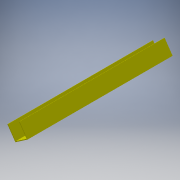
# Autodesk Inventor part: 2018 Concept Hook
Saved by Autodesk Inventor 2018 (Build 220112000, 112)
## iProperties
Created: 2018-01-18
Part Number: 2018 Concept Hook
Material: Generic
Document SubType Name: Modeling
Designer: Apple
Density: 1 g/cm^3
Appearance: Default
Author: Apple
Autodesk Inventor part; units mm, degrees
ref_plane "YZ Plane" through (0, 0, 0) normal (1, 0, 0) x (0, 1, 0)
ref_plane "XZ Plane" through (0, 0, 0) normal (0, 1, 0) x (-1, 0, 0)
ref_plane "XY Plane" through (0, 0, 0) normal (0, 0, 1) x (1, 0, 0)
sketch "Sketch1" plane through (0, 0, 0) normal (0, 0, 1) x (1, 0, 0)
  line L0 (39.103593, 49.524364) -> (75.147046, -2.754882)
  line L1 (75.147046, -2.754882) -> (22.8678, -38.798334)
  line L2 (22.8678, -38.798334) -> (-13.175652, 13.480911)
  line L3 (41.717556, 51.326537) -> (79.563181, -3.566671)
  line L4 (79.563181, -3.566671) -> (22.056011, -43.214469)
  line L5 (22.056011, -43.214469) -> (-15.789615, 11.678739)
  line L6 (-13.175652, 13.480911) -> (-15.789615, 11.678739)
  line L7 (41.717556, 51.326537) -> (39.103593, 49.524364)
  point P0 (0, 0)
  dimension "d0" = 63.5
  dimension "d1" = 63.5
  dimension "d2" = 63.5
  dimension "d3" = 3.175
  constraints: 16 end point, 4 perpendicular, 1 collinear, 2 other
  measures "d0" distance of L0.end L1.end
  measures "d1" distance of L1.end L2.end
  measures "d2" distance of L0.start L0.end
  measures "d3" distance between parallel lines of L0 L3
extrude "Extrusion1" add sketch "Sketch1" along normal blind 685.8
sketch "Sketch2" plane through (22.056011, -43.214469, 0) normal (-0.8232952, -0.5676134, 0) x (0, 0, 1)
  line L0 (0, 66.675) -> (0, 0)
  line L1 (0, 0) -> (685.8, 0)
  line L2 (685.8, 66.675) -> (685.8, 0)
  line L3 (0, 66.675) -> (685.8, 66.675)
  ellipse E0 centre (543.646569, 86.966998) end of major axis (522.564569, 86.966998) minor radius 21.081502
  line L4 (0, 3.175) -> (685.8, 3.175)
  line L5 (568.740496, 20.590277) -> (590.230156, 66.675)
  line L6 (0, 66.675) -> (685.8, 66.675)
  line L7 (466.695327, 66.675) -> (590.230156, 66.675)
  line L8 (508, 66.675) -> (177.8, 66.675) construction
  line L9 (177.8, 20.619453) -> (508, 20.619453) construction
  line L10 (508, 20.619453) -> (558.8, 20.619453) construction
  line L11 (558.8, 20.619453) -> (558.8, 66.675) construction
  line L12 (558.8, 66.675) -> (508, 66.675) construction
  line L13 (508, 66.675) -> (508, 20.619453) construction
  line L14 (466.695327, 66.675) -> (488.777383, 20.357192)
  arc A0 (488.653893, 20.619453) -> (516.003988, 3.175) centre (516.003988, 33.3375) ccw
  line L15 (541.403988, 3.175) -> (516.003988, 3.175)
  line L16 (0, 3.175) -> (685.8, 3.175)
  arc A1 (541.403988, 3.175) -> (568.740496, 20.590277) centre (541.403988, 33.3375) ccw
  line L17 (342.9, 3.175) -> (342.9, 66.675) construction
  line L18 (117.059504, 20.590277) -> (95.569844, 66.675)
  line L19 (219.104673, 66.675) -> (95.569844, 66.675)
  line L20 (177.8, 20.619453) -> (127, 20.619453) construction
  line L21 (127, 20.619453) -> (127, 66.675) construction
  line L22 (127, 66.675) -> (177.8, 66.675) construction
  line L23 (177.8, 66.675) -> (177.8, 20.619453) construction
  line L24 (219.104673, 66.675) -> (197.022617, 20.357192)
  arc A2 (169.796012, 3.175) -> (197.146107, 20.619453) centre (169.796012, 33.3375) ccw
  line L25 (144.396012, 3.175) -> (169.796012, 3.175)
  arc A3 (117.059504, 20.590277) -> (144.396012, 3.175) centre (144.396012, 33.3375) ccw
  point P0 (0, 48.097553)
  point P1 (342.9, 20.619453)
  point P2 (142.153431, 86.966998)
  point P3 (177.8, 66.675)
  dimension "d6" = 65
  dimension "d8" = 144.39601
  dimension "d10" = 330.2
  dimension "d11" = 50.8
  dimension "d14" = 25.4
  constraints: 38 end point, 14 symmetric about line, 10 point on circle, 9 point on line, 4 centre point, 4 tangent, 3 midpoint, 3 parallel, 2 horizontal, 1 collinear, 1 perpendicular, 1 vertical alignment, 3 other
  measures "d6" angle of L3 L5
  measures "d8" distance from line of L2 A1.centre
  measures "d10" distance of L9.start L9.end
  measures "d11" distance of L9.end L10.end
  measures "d14" distance of A0.centre A1.centre
extrude "Extrusion2" cut sketch "Sketch2" against normal blind 6.35 contours L3 L24 A2 L4 A3 L18 | L3 E0 L5 A1 L4 A0 L14 | L3 E0 picked at (543.004371, 66.441237)
body "Solid1"
